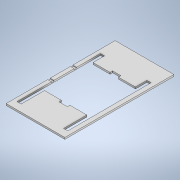
# Autodesk Inventor part: top_part
Saved by Autodesk Inventor 2020 (Build 240168000, 168)
## iProperties
Created: 2019-12-27
Part Number: top_part
Material: Générique
Document SubType Name: Modeling
Designer: damien
Density: 1 g/cm^3
Appearance: Par défaut
Author: damien
Autodesk Inventor part; units mm, degrees
ref_plane "YZ Plane" through (0, 0, 0) normal (1, 0, 0) x (0, 1, 0)
ref_plane "XZ Plane" through (0, 0, 0) normal (0, 1, 0) x (-1, 0, 0)
ref_plane "XY Plane" through (0, 0, 0) normal (0, 0, 1) x (1, 0, 0)
sketch "Esquisse1" plane through (0, 0, 0) normal (0, 1, 0) x (-1, 0, 0)
  line L0 (-350, -650) -> (350, -650)
  line L1 (350, -650) -> (350, 650)
  line L2 (350, 650) -> (-350, 650)
  line L3 (-350, 650) -> (-350, -650)
  line L4 (-350, -650) -> (350, 650) construction
  line L5 (350, -650) -> (-350, 650) construction
  point P0 (0, 0)
  dimension "d0" = 1300
  dimension "d1" = 700
  constraints: 12 end point, 2 midpoint, 2 parallel, 1 horizontal, 1 perpendicular
  measures "d0" distance of L0.end L1.end
  measures "d1" distance of L1.end L2.end
extrude "Extrusion1" add sketch "Esquisse1" along normal blind 20.7
sketch "Esquisse2" plane through (0, 20.7, 0) normal (0, 1, 0) x (1, 0, 0)
  line L0 (-305, -565.5) -> (-305, 429.5)
  line L1 (-305, 429.5) -> (-255, 429.5)
  line L2 (-255, 429.5) -> (-255, 292.5)
  line L3 (-255, 292.5) -> (250, 292.5)
  line L4 (250, 292.5) -> (250, 429.5)
  line L5 (250, 429.5) -> (300, 429.5)
  line L6 (300, 429.5) -> (300, -565.5)
  line L7 (300, -565.5) -> (250, -565.5)
  line L8 (250, -565.5) -> (250, -287.5)
  line L9 (250, -287.5) -> (-255, -287.5)
  line L10 (-255, -287.5) -> (-255, -565.5)
  line L11 (-255, -565.5) -> (-305, -565.5)
  line L12 (350, -650) -> (350, 650) projected
  line L13 (350, 0) -> (300, -68) construction
  line L14 (-350, 650) -> (-350, -650) projected
  line L15 (-350, -650) -> (350, -650) projected
  point P0 (0, 0)
  dimension "d4" = 995
  dimension "d5" = 50
  dimension "d6" = 605
  dimension "d7" = 580
  dimension "d8" = 137
  dimension "d9" = 50
  dimension "d10" = 84.5
  constraints: 26 end point, 7 perpendicular, 6 point on line, 2 equal length, 2 midpoint, 2 vertical
  measures "d4" distance of L5.end L6.end
  measures "d5" distance of L6.end L7.end
  measures "d6" distance between parallel lines of L0 L6
  measures "d7" distance between parallel lines of L3 L9
  measures "d8" distance of L3.end L4.end
  measures "d9" distance between parallel lines of L12 L6
  measures "d10" distance between parallel lines of L15 L11
extrude "Extrusion2" cut sketch "Esquisse2" against normal blind 21.1
sketch "Esquisse3" plane through (-350, 0, 650) normal (1, 0, 0) x (0, 0, -1)
  line L0 (84.5, 20.7) -> (1079.5, 20.7) projected
  line L1 (495, 20.7) -> (525, 20.7)
  line L2 (525, 20.7) -> (525, 10.7)
  line L3 (525, 10.7) -> (495, 10.7)
  line L4 (495, 10.7) -> (495, 20.7)
  line L5 (0, 0) -> (0, 20.7) projected
  line L6 (765, 20.7) -> (795, 20.7)
  line L7 (795, 20.7) -> (795, 10.7)
  line L8 (795, 10.7) -> (765, 10.7)
  line L9 (765, 10.7) -> (765, 20.7)
  point P0 (650, 0)
  dimension "d13" = 495
  dimension "d14" = 30
  dimension "d15" = 10
  dimension "d16" = 240
  dimension "d17" = 30
  constraints: 16 end point, 4 parallel, 2 horizontal, 2 perpendicular, 2 point on line, 1 collinear
  measures "d13" distance from line of L5 L1.start
  measures "d14" distance of L2.end L3.end
  measures "d15" distance of L1.end L2.end
  measures "d16" distance between parallel lines of L9 L2
  measures "d17" distance of L7.end L8.end
extrude "Extrusion3" cut sketch "Esquisse3" along normal blind 100
sketch "Esquisse4" plane through (0, 20.7, 0) normal (0, 1, 0) x (1, 0, 0)
  line L0 (250, 292.5) -> (-255, 292.5) projected
  line L1 (-52.5, 292.5) -> (47.5, 292.5)
  line L2 (47.5, 292.5) -> (47.5, 322.5)
  line L3 (47.5, 322.5) -> (-52.5, 322.5)
  line L4 (-52.5, 322.5) -> (-52.5, 292.5)
  line L5 (-255, -287.5) -> (250, -287.5) projected
  line L6 (-52.5, -287.5) -> (47.5, -287.5)
  line L7 (47.5, -287.5) -> (47.5, -317.5)
  line L8 (47.5, -317.5) -> (-52.5, -317.5)
  line L9 (-52.5, -317.5) -> (-52.5, -287.5)
  line L10 (-255, 429.5) -> (-255, 292.5) projected
  line L11 (250, 292.5) -> (250, 429.5) projected
  point P0 (0, 0)
  point P1 (47.5, -287.5)
  dimension "d20" = 30
  dimension "d21" = 100
  dimension "d22" = 202.5
  dimension "d23" = 202.5
  constraints: 16 end point, 4 parallel, 4 point on line, 2 horizontal, 2 perpendicular, 1 collinear
  measures "d20" distance of L6.end L7.end
  measures "d21" distance of L2.end L3.end
  measures "d22" distance between parallel lines of L10 L4
  measures "d23" distance between parallel lines of L11 L2
extrude "Extrusion4" cut sketch "Esquisse4" against normal blind 100
fillet "Congé1" radius 2 8 edges at (47.5, 10.35, -322.5) (47.5, 10.35, -292.5) (-52.5, 10.35, -322.5) (-52.5, 10.35, -292.5) (-52.5, 10.35, 287.5) (-52.5, 10.35, 317.5) (47.5, 10.35, 317.5) (47.5, 10.35, 287.5)
